Autodesk Fusion 360 part; units mm, degrees
(part 20 of 40)
  line L1487 (51.4118, 42.8386) -> (51.5684, 42.8818) construction
  line L1488 (51.5684, 42.8818) -> (51.7255, 42.9241) construction
  line L1489 (51.7255, 42.9241) -> (51.883, 42.9656) construction
  line L1490 (51.883, 42.9656) -> (52.0409, 43.0063) construction
  line L1491 (52.0409, 43.0063) -> (52.1993, 43.0461) construction
  line L1492 (52.1993, 43.0461) -> (52.3581, 43.085) construction
  line L1493 (52.3581, 43.085) -> (52.5173, 43.1231) construction
  line L1494 (52.5173, 43.1231) -> (52.6769, 43.1604) construction
  line L1495 (52.6769, 43.1604) -> (52.8369, 43.1969) construction
  line L1496 (52.8369, 43.1969) -> (52.9973, 43.2326) construction
  line L1497 (52.9973, 43.2326) -> (53.1581, 43.2674) construction
  line L1498 (53.1581, 43.2674) -> (53.3193, 43.3015) construction
  line L1499 (53.3193, 43.3015) -> (53.4809, 43.3347) construction
  line L1500 (53.4809, 43.3347) -> (53.6428, 43.3672) construction
  line L1501 (53.6428, 43.3672) -> (53.8051, 43.3988) construction
  line L1502 (53.8051, 43.3988) -> (53.9677, 43.4297) construction
  line L1503 (53.9677, 43.4297) -> (54.1307, 43.4597) construction
  line L1504 (54.1307, 43.4597) -> (54.294, 43.489) construction
  line L1505 (54.294, 43.489) -> (54.4577, 43.5175) construction
  line L1506 (54.4577, 43.5175) -> (54.6217, 43.5453) construction
  line L1507 (54.6217, 43.5453) -> (54.7861, 43.5723) construction
  line L1508 (54.7861, 43.5723) -> (54.9508, 43.5984) construction
  line L1509 (54.9508, 43.5984) -> (55.1158, 43.6239) construction
  line L1510 (55.1158, 43.6239) -> (55.2811, 43.6486) construction
  line L1511 (55.2811, 43.6486) -> (55.4467, 43.6725) construction
  line L1512 (55.4467, 43.6725) -> (55.6126, 43.6956) construction
  line L1513 (55.6126, 43.6956) -> (55.7789, 43.718) construction
  line L1514 (55.7789, 43.718) -> (55.9454, 43.7397) construction
  line L1515 (55.9454, 43.7397) -> (56.1122, 43.7606) construction
  line L1516 (56.1122, 43.7606) -> (56.2459, 43.7767) construction
  line L1517 (56.2459, 43.7767) -> (56.3463, 43.7885) construction
  line L1518 (56.3463, 43.7885) -> (56.4133, 43.7962) construction
  line L1519 (56.4133, 43.7962) -> (56.4469, 43.8) construction
  line L1520 (56.0345, -24.1948) -> (56.0628, -24.2071) construction
  line L1521 (56.0628, -24.2071) -> (56.1198, -24.2308) construction
  line L1522 (56.1198, -24.2308) -> (56.2062, -24.264) construction
  line L1523 (56.2062, -24.264) -> (56.3229, -24.3039) construction
  line L1524 (56.3229, -24.3039) -> (56.4711, -24.3478) construction
  line L1525 (56.4711, -24.3478) -> (56.6208, -24.3873) construction
  line L1526 (56.6208, -24.3873) -> (56.7714, -24.4241) construction
  line L1527 (56.7714, -24.4241) -> (56.9226, -24.4595) construction
  line L1528 (56.9226, -24.4595) -> (57.0741, -24.494) construction
  line L1529 (57.0741, -24.494) -> (57.226, -24.5274) construction
  line L1530 (57.226, -24.5274) -> (57.3783, -24.5594) construction
  line L1531 (57.3783, -24.5594) -> (57.5312, -24.5896) construction
  line L1532 (57.5312, -24.5896) -> (57.6848, -24.6176) construction
  line L1533 (57.6848, -24.6176) -> (57.8391, -24.6435) construction
  line L1534 (57.8391, -24.6435) -> (57.994, -24.6674) construction
  line L1535 (57.994, -24.6674) -> (58.1494, -24.6897) construction
  line L1536 (58.1494, -24.6897) -> (58.3052, -24.7105) construction
  line L1537 (58.3052, -24.7105) -> (58.4614, -24.7301) construction
  line L1538 (58.4614, -24.7301) -> (58.6179, -24.7485) construction
  line L1539 (58.6179, -24.7485) -> (58.7747, -24.7658) construction
  line L1540 (58.7747, -24.7658) -> (58.9318, -24.7818) construction
  line L1541 (58.9318, -24.7818) -> (59.0893, -24.7965) construction
  line L1542 (59.0893, -24.7965) -> (59.2471, -24.8098) construction
  line L1543 (59.2471, -24.8098) -> (59.4053, -24.8218) construction
  line L1544 (59.4053, -24.8218) -> (59.5638, -24.8325) construction
  line L1545 (59.5638, -24.8325) -> (59.7226, -24.842) construction
  line L1546 (59.7226, -24.842) -> (59.8817, -24.8504) construction
  line L1547 (59.8817, -24.8504) -> (60.0411, -24.8577) construction
  line L1548 (60.0411, -24.8577) -> (60.2007, -24.8638) construction
  line L1549 (60.2007, -24.8638) -> (60.3605, -24.8689) construction
  line L1550 (60.3605, -24.8689) -> (60.5206, -24.8729) construction
  line L1551 (60.5206, -24.8729) -> (60.6809, -24.8757) construction
  line L1552 (60.6809, -24.8757) -> (60.8415, -24.8776) construction
  line L1553 (60.8415, -24.8776) -> (61.0023, -24.8783) construction
  line L1554 (61.0023, -24.8783) -> (61.1633, -24.878) construction
  line L1555 (61.1633, -24.878) -> (61.3245, -24.8766) construction
  line L1556 (61.3245, -24.8766) -> (61.4859, -24.8742) construction
  line L1557 (61.4859, -24.8742) -> (61.6475, -24.8708) construction
  line L1558 (61.6475, -24.8708) -> (61.8093, -24.8665) construction
  line L1559 (61.8093, -24.8665) -> (61.9712, -24.8611) construction
  line L1560 (61.9712, -24.8611) -> (62.1334, -24.8548) construction
  line L1561 (62.1334, -24.8548) -> (62.2957, -24.8475) construction
  line L1562 (62.2957, -24.8475) -> (62.4581, -24.8392) construction
  line L1563 (62.4581, -24.8392) -> (62.6207, -24.83) construction
  line L1564 (62.6207, -24.83) -> (62.7835, -24.8199) construction
  line L1565 (62.7835, -24.8199) -> (62.9464, -24.8088) construction
  line L1566 (62.9464, -24.8088) -> (63.1095, -24.7967) construction
  line L1567 (63.1095, -24.7967) -> (63.2727, -24.7838) construction
  line L1568 (63.2727, -24.7838) -> (63.436, -24.77) construction
  line L1569 (63.436, -24.77) -> (63.5995, -24.7552) construction
  line L1570 (63.5995, -24.7552) -> (63.7631, -24.7396) construction
  line L1571 (63.7631, -24.7396) -> (63.9268, -24.723) construction
  line L1572 (63.9268, -24.723) -> (64.0906, -24.7056) construction
  line L1573 (64.0906, -24.7056) -> (64.2545, -24.6873) construction
  line L1574 (64.2545, -24.6873) -> (64.4185, -24.6681) construction
  line L1575 (64.4185, -24.6681) -> (64.5826, -24.648) construction
  line L1576 (64.5826, -24.648) -> (64.7468, -24.6271) construction
  line L1577 (64.7468, -24.6271) -> (64.9111, -24.6054) construction
  line L1578 (64.9111, -24.6054) -> (65.0755, -24.5828) construction
  line L1579 (65.0755, -24.5828) -> (65.24, -24.5593) construction
  line L1580 (65.24, -24.5593) -> (65.4046, -24.535) construction
  line L1581 (65.4046, -24.535) -> (65.5692, -24.5098) construction
  line L1582 (65.5692, -24.5098) -> (65.734, -24.4839) construction
  line L1583 (65.734, -24.4839) -> (65.8987, -24.4571) construction
  line L1584 (65.8987, -24.4571) -> (66.0636, -24.4294) construction
  line L1585 (66.0636, -24.4294) -> (66.2285, -24.401) construction
  line L1586 (66.2285, -24.401) -> (66.3935, -24.3718) construction
  line L1587 (66.3935, -24.3718) -> (66.5585, -24.3417) construction
  line L1588 (66.5585, -24.3417) -> (66.7236, -24.3108) construction
  line L1589 (66.7236, -24.3108) -> (66.8887, -24.2792) construction
  line L1590 (66.8887, -24.2792) -> (67.0208, -24.2532) construction
  line L1591 (67.0208, -24.2532) -> (67.1199, -24.2334) construction
  line L1592 (67.1199, -24.2334) -> (67.186, -24.22) construction
  line L1593 (67.186, -24.22) -> (67.2191, -24.2132) construction
  line L1594 (52.5103, -31.1115) -> (52.5368, -31.1272) construction
  line L1595 (52.5368, -31.1272) -> (52.5895, -31.1594) construction
  line L1596 (52.5895, -31.1594) -> (52.6672, -31.2097) construction
  line L1597 (52.6672, -31.2097) -> (52.7681, -31.2807) construction
  line L1598 (52.7681, -31.2807) -> (52.8906, -31.3748) construction
  line L1599 (52.8906, -31.3748) -> (53.0106, -31.4727) construction
  line L1600 (53.0106, -31.4727) -> (53.1289, -31.5729) construction
  line L1601 (53.1289, -31.5729) -> (53.2464, -31.6744) construction
  line L1602 (53.2464, -31.6744) -> (53.3634, -31.7767) construction
  line L1603 (53.3634, -31.7767) -> (53.4797, -31.88) construction
  line L1604 (53.4797, -31.88) -> (53.5951, -31.9844) construction
  line L1605 (53.5951, -31.9844) -> (53.7094, -32.0903) construction
  line L1606 (53.7094, -32.0903) -> (53.8224, -32.1981) construction
  line L1607 (53.8224, -32.1981) -> (53.934, -32.3077) construction
  line L1608 (53.934, -32.3077) -> (54.0444, -32.419) construction
  line L1609 (54.0444, -32.419) -> (54.1537, -32.5316) construction
  line L1610 (54.1537, -32.5316) -> (54.2622, -32.6455) construction
  line L1611 (54.2622, -32.6455) -> (54.3698, -32.7603) construction
  line L1612 (54.3698, -32.7603) -> (54.4767, -32.876) construction
  line L1613 (54.4767, -32.876) -> (54.5828, -32.9927) construction
  line L1614 (54.5828, -32.9927) -> (54.6881, -33.1105) construction
  line L1615 (54.6881, -33.1105) -> (54.7926, -33.2292) construction
  line L1616 (54.7926, -33.2292) -> (54.8961, -33.3491) construction
  line L1617 (54.8961, -33.3491) -> (54.9988, -33.47) construction
  line L1618 (54.9988, -33.47) -> (55.1007, -33.5919) construction
  line L1619 (55.1007, -33.5919) -> (55.2017, -33.7148) construction
  line L1620 (55.2017, -33.7148) -> (55.302, -33.8386) construction
  line L1621 (55.302, -33.8386) -> (55.4015, -33.9633) construction
  line L1622 (55.4015, -33.9633) -> (55.5003, -34.0888) construction
  line L1623 (55.5003, -34.0888) -> (55.5984, -34.2151) construction
  line L1624 (55.5984, -34.2151) -> (55.6957, -34.3423) construction
  line L1625 (55.6957, -34.3423) -> (55.7923, -34.4703) construction
  line L1626 (55.7923, -34.4703) -> (55.8881, -34.5991) construction
  line L1627 (55.8881, -34.5991) -> (55.9832, -34.7288) construction
  line L1628 (55.9832, -34.7288) -> (56.0776, -34.8592) construction
  line L1629 (56.0776, -34.8592) -> (56.1712, -34.9905) construction
  line L1630 (56.1712, -34.9905) -> (56.2642, -35.1224) construction
  line L1631 (56.2642, -35.1224) -> (56.3564, -35.2552) construction
  line L1632 (56.3564, -35.2552) -> (56.448, -35.3886) construction
  line L1633 (56.448, -35.3886) -> (56.5388, -35.5228) construction
  line L1634 (56.5388, -35.5228) -> (56.629, -35.6577) construction
  line L1635 (56.629, -35.6577) -> (56.7185, -35.7933) construction
  line L1636 (56.7185, -35.7933) -> (56.8073, -35.9295) construction
  line L1637 (56.8073, -35.9295) -> (56.8955, -36.0665) construction
  line L1638 (56.8955, -36.0665) -> (56.9829, -36.2042) construction
  line L1639 (56.9829, -36.2042) -> (57.0697, -36.3425) construction
  line L1640 (57.0697, -36.3425) -> (57.1558, -36.4815) construction
  line L1641 (57.1558, -36.4815) -> (57.2413, -36.6211) construction
  line L1642 (57.2413, -36.6211) -> (57.3261, -36.7614) construction
  line L1643 (57.3261, -36.7614) -> (57.4102, -36.9023) construction
  line L1644 (57.4102, -36.9023) -> (57.4937, -37.0438) construction
  line L1645 (57.4937, -37.0438) -> (57.5765, -37.186) construction
  line L1646 (57.5765, -37.186) -> (57.6587, -37.3288) construction
  line L1647 (57.6587, -37.3288) -> (57.7403, -37.4721) construction
  line L1648 (57.7403, -37.4721) -> (57.8212, -37.6161) construction
  line L1649 (57.8212, -37.6161) -> (57.9014, -37.7607) construction
  line L1650 (57.9014, -37.7607) -> (57.981, -37.9058) construction
  line L1651 (57.981, -37.9058) -> (58.06, -38.0515) construction
  line L1652 (58.06, -38.0515) -> (58.1383, -38.1978) construction
  line L1653 (58.1383, -38.1978) -> (58.216, -38.3447) construction
  line L1654 (58.216, -38.3447) -> (58.2931, -38.4921) construction
  line L1655 (58.2931, -38.4921) -> (58.3695, -38.6401) construction
  line L1656 (58.3695, -38.6401) -> (58.4453, -38.7886) construction
  line L1657 (58.4453, -38.7886) -> (58.5205, -38.9377) construction
  line L1658 (58.5205, -38.9377) -> (58.595, -39.0873) construction
  line L1659 (58.595, -39.0873) -> (58.669, -39.2374) construction
  line L1660 (58.669, -39.2374) -> (58.7423, -39.3881) construction
  line L1661 (58.7423, -39.3881) -> (58.8149, -39.5393) construction
  line L1662 (58.8149, -39.5393) -> (58.887, -39.6909) construction
  line L1663 (58.887, -39.6909) -> (58.9584, -39.8431) construction
  line L1664 (58.9584, -39.8431) -> (59.0151, -39.9653) construction
  line L1665 (59.0151, -39.9653) -> (59.0573, -40.0572) construction
  line L1666 (59.0573, -40.0572) -> (59.0853, -40.1185) construction
  line L1667 (59.0853, -40.1185) -> (59.0993, -40.1492) construction
  line L1668 (-13.3622, -59.5542) -> (-13.369, -59.5843) construction
  line L1669 (-13.369, -59.5843) -> (-13.3833, -59.6444) construction
  line L1670 (-13.3833, -59.6444) -> (-13.4071, -59.7338) construction
  line L1671 (-13.4071, -59.7338) -> (-13.4435, -59.8517) construction
  line L1672 (-13.4435, -59.8517) -> (-13.4951, -59.9973) construction
  line L1673 (-13.4951, -59.9973) -> (-13.5511, -60.1416) construction
  line L1674 (-13.5511, -60.1416) -> (-13.6099, -60.2852) construction
  line L1675 (-13.6099, -60.2852) -> (-13.6701, -60.4283) construction
  line L1676 (-13.6701, -60.4283) -> (-13.7313, -60.5711) construction
  line L1677 (-13.7313, -60.5711) -> (-13.7935, -60.7136) construction
  line L1678 (-13.7935, -60.7136) -> (-13.8571, -60.8557) construction
  line L1679 (-13.8571, -60.8557) -> (-13.9226, -60.9971) construction
  line L1680 (-13.9226, -60.9971) -> (-13.9902, -61.1379) construction
  line L1681 (-13.9902, -61.1379) -> (-14.06, -61.2779) construction
  line L1682 (-14.06, -61.2779) -> (-14.1316, -61.4173) construction
  line L1683 (-14.1316, -61.4173) -> (-14.205, -61.5561) construction
  line L1684 (-14.205, -61.5561) -> (-14.2797, -61.6944) construction
  line L1685 (-14.2797, -61.6944) -> (-14.3557, -61.8322) construction
  line L1686 (-14.3557, -61.8322) -> (-14.4327, -61.9697) construction
  line L1687 (-14.4327, -61.9697) -> (-14.5109, -62.1067) construction
  line L1688 (-14.5109, -62.1067) -> (-14.5904, -62.2432) construction
  line L1689 (-14.5904, -62.2432) -> (-14.6711, -62.3792) construction
  line L1690 (-14.6711, -62.3792) -> (-14.753, -62.5148) construction
  line L1691 (-14.753, -62.5148) -> (-14.8363, -62.6498) construction
  line L1692 (-14.8363, -62.6498) -> (-14.9208, -62.7843) construction
  line L1693 (-14.9208, -62.7843) -> (-15.0064, -62.9184) construction
  line L1694 (-15.0064, -62.9184) -> (-15.0932, -63.052) construction
  line L1695 (-15.0932, -63.052) -> (-15.181, -63.1852) construction
  line L1696 (-15.181, -63.1852) -> (-15.2698, -63.318) construction
  line L1697 (-15.2698, -63.318) -> (-15.3597, -63.4503) construction
  line L1698 (-15.3597, -63.4503) -> (-15.4506, -63.5821) construction
  line L1699 (-15.4506, -63.5821) -> (-15.5425, -63.7135) construction
  line L1700 (-15.5425, -63.7135) -> (-15.6354, -63.8445) construction
  line L1701 (-15.6354, -63.8445) -> (-15.7293, -63.975) construction
  line L1702 (-15.7293, -63.975) -> (-15.8242, -64.105) construction
  line L1703 (-15.8242, -64.105) -> (-15.92, -64.2346) construction
  line L1704 (-15.92, -64.2346) -> (-16.0168, -64.3638) construction
  line L1705 (-16.0168, -64.3638) -> (-16.1146, -64.4926) construction
  line L1706 (-16.1146, -64.4926) -> (-16.2132, -64.6209) construction
  line L1707 (-16.2132, -64.6209) -> (-16.3127, -64.7488) construction
  line L1708 (-16.3127, -64.7488) -> (-16.4131, -64.8762) construction
  line L1709 (-16.4131, -64.8762) -> (-16.5144, -65.0032) construction
  line L1710 (-16.5144, -65.0032) -> (-16.6166, -65.1298) construction
  line L1711 (-16.6166, -65.1298) -> (-16.7196, -65.256) construction
  line L1712 (-16.7196, -65.256) -> (-16.8235, -65.3817) construction
  line L1713 (-16.8235, -65.3817) -> (-16.9283, -65.507) construction
  line L1714 (-16.9283, -65.507) -> (-17.0338, -65.6318) construction
  line L1715 (-17.0338, -65.6318) -> (-17.1402, -65.7562) construction
  line L1716 (-17.1402, -65.7562) -> (-17.2474, -65.8802) construction
  line L1717 (-17.2474, -65.8802) -> (-17.3555, -66.0038) construction
  line L1718 (-17.3555, -66.0038) -> (-17.4643, -66.1269) construction
  line L1719 (-17.4643, -66.1269) -> (-17.5739, -66.2497) construction
  line L1720 (-17.5739, -66.2497) -> (-17.6842, -66.3719) construction
  line L1721 (-17.6842, -66.3719) -> (-17.7954, -66.4938) construction
  line L1722 (-17.7954, -66.4938) -> (-17.9073, -66.6152) construction
  line L1723 (-17.9073, -66.6152) -> (-18.02, -66.7362) construction
  line L1724 (-18.02, -66.7362) -> (-18.1335, -66.8568) construction
  line L1725 (-18.1335, -66.8568) -> (-18.2477, -66.9769) construction
  line L1726 (-18.2477, -66.9769) -> (-18.3626, -67.0966) construction
  line L1727 (-18.3626, -67.0966) -> (-18.4782, -67.2159) construction
  line L1728 (-18.4782, -67.2159) -> (-18.5946, -67.3347) construction
  line L1729 (-18.5946, -67.3347) -> (-18.7118, -67.4531) construction
  line L1730 (-18.7118, -67.4531) -> (-18.8296, -67.5711) construction
  line L1731 (-18.8296, -67.5711) -> (-18.9481, -67.6887) construction
  line L1732 (-18.9481, -67.6887) -> (-19.0674, -67.8058) construction
  line L1733 (-19.0674, -67.8058) -> (-19.1873, -67.9225) construction
  line L1734 (-19.1873, -67.9225) -> (-19.3079, -68.0388) construction
  line L1735 (-19.3079, -68.0388) -> (-19.4293, -68.1546) construction
  line L1736 (-19.4293, -68.1546) -> (-19.5512, -68.27) construction
  line L1737 (-19.5512, -68.27) -> (-19.6739, -68.385) construction
  line L1738 (-19.6739, -68.385) -> (-19.7726, -68.4767) construction
  line L1739 (-19.7726, -68.4767) -> (-19.8469, -68.5452) construction
  line L1740 (-19.8469, -68.5452) -> (-19.8966, -68.5908) construction
  line L1741 (-19.8966, -68.5908) -> (-19.9215, -68.6136) construction
  line L1742 (-45.8153, 40.3263) -> (-45.8385, 40.3467) construction
  line L1743 (-45.8385, 40.3467) -> (-45.8854, 40.3868) construction
  line L1744 (-45.8854, 40.3868) -> (-45.9573, 40.4451) construction
  line L1745 (-45.9573, 40.4451) -> (-46.056, 40.5192) construction
  line L1746 (-46.056, 40.5192) -> (-46.1833, 40.6066) construction
  line L1747 (-46.1833, 40.6066) -> (-46.3135, 40.6904) construction
  line L1748 (-46.3135, 40.6904) -> (-46.4454, 40.772) construction
  line L1749 (-46.4454, 40.772) -> (-46.5782, 40.8524) construction
  line L1750 (-46.5782, 40.8524) -> (-46.7117, 40.932) construction
  line L1751 (-46.7117, 40.932) -> (-46.8458, 41.0107) construction
  line L1752 (-46.8458, 41.0107) -> (-46.9807, 41.0883) construction
  line L1753 (-46.9807, 41.0883) -> (-47.1168, 41.1642) construction
  line L1754 (-47.1168, 41.1642) -> (-47.2543, 41.2383) construction
  line L1755 (-47.2543, 41.2383) -> (-47.393, 41.3106) construction
  line L1756 (-47.393, 41.3106) -> (-47.5329, 41.3813) construction
  line L1757 (-47.5329, 41.3813) -> (-47.6738, 41.4504) construction
  line L1758 (-47.6738, 41.4504) -> (-47.8156, 41.5184) construction
  line L1759 (-47.8156, 41.5184) -> (-47.9581, 41.5853) construction
  line L1760 (-47.9581, 41.5853) -> (-48.1012, 41.6512) construction
  line L1761 (-48.1012, 41.6512) -> (-48.245, 41.716) construction
  line L1762 (-48.245, 41.716) -> (-48.3895, 41.7798) construction
  line L1763 (-48.3895, 41.7798) -> (-48.5347, 41.8424) construction
  line L1764 (-48.5347, 41.8424) -> (-48.6807, 41.9039) construction
  line L1765 (-48.6807, 41.9039) -> (-48.8274, 41.9642) construction
  line L1766 (-48.8274, 41.9642) -> (-48.9749, 42.0234) construction
  line L1767 (-48.9749, 42.0234) -> (-49.123, 42.0815) construction
  line L1768 (-49.123, 42.0815) -> (-49.2717, 42.1386) construction
  line L1769 (-49.2717, 42.1386) -> (-49.421, 42.1947) construction
  line L1770 (-49.421, 42.1947) -> (-49.5709, 42.2499) construction
  line L1771 (-49.5709, 42.2499) -> (-49.7214, 42.3041) construction
  line L1772 (-49.7214, 42.3041) -> (-49.8724, 42.3574) construction
  line L1773 (-49.8724, 42.3574) -> (-50.024, 42.4097) construction
  line L1774 (-50.024, 42.4097) -> (-50.1761, 42.461) construction
  line L1775 (-50.1761, 42.461) -> (-50.3288, 42.5114) construction
  line L1776 (-50.3288, 42.5114) -> (-50.482, 42.5608) construction
  line L1777 (-50.482, 42.5608) -> (-50.6358, 42.6094) construction
  line L1778 (-50.6358, 42.6094) -> (-50.79, 42.657) construction
  line L1779 (-50.79, 42.657) -> (-50.9447, 42.7037) construction
  line L1780 (-50.9447, 42.7037) -> (-51.0999, 42.7495) construction
  line L1781 (-51.0999, 42.7495) -> (-51.2556, 42.7945) construction
  line L1782 (-51.2556, 42.7945) -> (-51.4118, 42.8386) construction
  line L1783 (-51.4118, 42.8386) -> (-51.5684, 42.8818) construction
  line L1784 (-51.5684, 42.8818) -> (-51.7255, 42.9241) construction
  line L1785 (-51.7255, 42.9241) -> (-51.883, 42.9656) construction
  line L1786 (-51.883, 42.9656) -> (-52.0409, 43.0063) construction
  line L1787 (-52.0409, 43.0063) -> (-52.1993, 43.0461) construction
  line L1788 (-52.1993, 43.0461) -> (-52.3581, 43.085) construction
  line L1789 (-52.3581, 43.085) -> (-52.5173, 43.1231) construction
  line L1790 (-52.5173, 43.1231) -> (-52.6769, 43.1604) construction
  line L1791 (-52.6769, 43.1604) -> (-52.8369, 43.1969) construction
  line L1792 (-52.8369, 43.1969) -> (-52.9973, 43.2326) construction
  line L1793 (-52.9973, 43.2326) -> (-53.1581, 43.2674) construction
  line L1794 (-53.1581, 43.2674) -> (-53.3193, 43.3015) construction
  line L1795 (-53.3193, 43.3015) -> (-53.4809, 43.3347) construction
  line L1796 (-53.4809, 43.3347) -> (-53.6428, 43.3672) construction
  line L1797 (-53.6428, 43.3672) -> (-53.8051, 43.3988) construction
  line L1798 (-53.8051, 43.3988) -> (-53.9677, 43.4297) construction
  line L1799 (-53.9677, 43.4297) -> (-54.1307, 43.4597) construction
  line L1800 (-54.1307, 43.4597) -> (-54.294, 43.489) construction
  line L1801 (-54.294, 43.489) -> (-54.4577, 43.5175) construction
  line L1802 (-54.4577, 43.5175) -> (-54.6217, 43.5453) construction
  line L1803 (-54.6217, 43.5453) -> (-54.7861, 43.5723) construction
  line L1804 (-54.7861, 43.5723) -> (-54.9508, 43.5984) construction
  line L1805 (-54.9508, 43.5984) -> (-55.1158, 43.6239) construction
  line L1806 (-55.1158, 43.6239) -> (-55.2811, 43.6486) construction
  line L1807 (-55.2811, 43.6486) -> (-55.4467, 43.6725) construction
  line L1808 (-55.4467, 43.6725) -> (-55.6126, 43.6956) construction
  line L1809 (-55.6126, 43.6956) -> (-55.7789, 43.718) construction
  line L1810 (-55.7789, 43.718) -> (-55.9454, 43.7397) construction
  line L1811 (-55.9454, 43.7397) -> (-56.1122, 43.7606) construction
  line L1812 (-56.1122, 43.7606) -> (-56.2459, 43.7767) construction
  line L1813 (-56.2459, 43.7767) -> (-56.3463, 43.7885) construction
  line L1814 (-56.3463, 43.7885) -> (-56.4133, 43.7962) construction
  line L1815 (-56.4133, 43.7962) -> (-56.4469, 43.8) construction
  line L1816 (59.5542, 13.3622) -> (59.5843, 13.369) construction
  line L1817 (59.5843, 13.369) -> (59.6444, 13.3833) construction
  line L1818 (59.6444, 13.3833) -> (59.7338, 13.4071) construction
  line L1819 (59.7338, 13.4071) -> (59.8517, 13.4435) construction
  line L1820 (59.8517, 13.4435) -> (59.9973, 13.4951) construction
  line L1821 (59.9973, 13.4951) -> (60.1416, 13.5511) construction
  line L1822 (60.1416, 13.5511) -> (60.2852, 13.6099) construction
  line L1823 (60.2852, 13.6099) -> (60.4283, 13.6701) construction
  line L1824 (60.4283, 13.6701) -> (60.5711, 13.7313) construction
  line L1825 (60.5711, 13.7313) -> (60.7136, 13.7935) construction
  line L1826 (60.7136, 13.7935) -> (60.8557, 13.8571) construction
  line L1827 (60.8557, 13.8571) -> (60.9971, 13.9226) construction
  line L1828 (60.9971, 13.9226) -> (61.1379, 13.9902) construction
  line L1829 (61.1379, 13.9902) -> (61.2779, 14.06) construction
  line L1830 (61.2779, 14.06) -> (61.4173, 14.1316) construction
  line L1831 (61.4173, 14.1316) -> (61.5561, 14.205) construction
  line L1832 (61.5561, 14.205) -> (61.6944, 14.2797) construction
  line L1833 (61.6944, 14.2797) -> (61.8322, 14.3557) construction
  line L1834 (61.8322, 14.3557) -> (61.9697, 14.4327) construction
  line L1835 (61.9697, 14.4327) -> (62.1067, 14.5109) construction
  line L1836 (62.1067, 14.5109) -> (62.2432, 14.5904) construction
  line L1837 (62.2432, 14.5904) -> (62.3792, 14.6711) construction
  line L1838 (62.3792, 14.6711) -> (62.5148, 14.753) construction
  line L1839 (62.5148, 14.753) -> (62.6498, 14.8363) construction
  line L1840 (62.6498, 14.8363) -> (62.7843, 14.9208) construction
  line L1841 (62.7843, 14.9208) -> (62.9184, 15.0064) construction
  line L1842 (62.9184, 15.0064) -> (63.052, 15.0932) construction
  line L1843 (63.052, 15.0932) -> (63.1852, 15.181) construction
  line L1844 (63.1852, 15.181) -> (63.318, 15.2698) construction
  line L1845 (63.318, 15.2698) -> (63.4503, 15.3597) construction
  line L1846 (63.4503, 15.3597) -> (63.5821, 15.4506) construction
  line L1847 (63.5821, 15.4506) -> (63.7135, 15.5425) construction
  line L1848 (63.7135, 15.5425) -> (63.8445, 15.6354) construction
  line L1849 (63.8445, 15.6354) -> (63.975, 15.7293) construction
  line L1850 (63.975, 15.7293) -> (64.105, 15.8242) construction
  line L1851 (64.105, 15.8242) -> (64.2346, 15.92) construction
  line L1852 (64.2346, 15.92) -> (64.3638, 16.0168) construction
  line L1853 (64.3638, 16.0168) -> (64.4926, 16.1146) construction
  line L1854 (64.4926, 16.1146) -> (64.6209, 16.2132) construction
  line L1855 (64.6209, 16.2132) -> (64.7488, 16.3127) construction
  line L1856 (64.7488, 16.3127) -> (64.8762, 16.4131) construction
  line L1857 (64.8762, 16.4131) -> (65.0032, 16.5144) construction
  line L1858 (65.0032, 16.5144) -> (65.1298, 16.6166) construction
  line L1859 (65.1298, 16.6166) -> (65.256, 16.7196) construction
  line L1860 (65.256, 16.7196) -> (65.3817, 16.8235) construction
  line L1861 (65.3817, 16.8235) -> (65.507, 16.9283) construction
  line L1862 (65.507, 16.9283) -> (65.6318, 17.0338) construction
  line L1863 (65.6318, 17.0338) -> (65.7562, 17.1402) construction
  line L1864 (65.7562, 17.1402) -> (65.8802, 17.2474) construction
  line L1865 (65.8802, 17.2474) -> (66.0038, 17.3555) construction
  line L1866 (66.0038, 17.3555) -> (66.1269, 17.4643) construction
  line L1867 (66.1269, 17.4643) -> (66.2497, 17.5739) construction
  line L1868 (66.2497, 17.5739) -> (66.3719, 17.6842) construction
  line L1869 (66.3719, 17.6842) -> (66.4938, 17.7954) construction
  line L1870 (66.4938, 17.7954) -> (66.6152, 17.9073) construction
  line L1871 (66.6152, 17.9073) -> (66.7362, 18.02) construction
  line L1872 (66.7362, 18.02) -> (66.8568, 18.1335) construction
  line L1873 (66.8568, 18.1335) -> (66.9769, 18.2477) construction
  line L1874 (66.9769, 18.2477) -> (67.0966, 18.3626) construction
  line L1875 (67.0966, 18.3626) -> (67.2159, 18.4782) construction
  line L1876 (67.2159, 18.4782) -> (67.3347, 18.5946) construction
  line L1877 (67.3347, 18.5946) -> (67.4531, 18.7118) construction
  line L1878 (67.4531, 18.7118) -> (67.5711, 18.8296) construction
  line L1879 (67.5711, 18.8296) -> (67.6887, 18.9481) construction
  line L1880 (67.6887, 18.9481) -> (67.8058, 19.0674) construction
  line L1881 (67.8058, 19.0674) -> (67.9225, 19.1873) construction
  line L1882 (67.9225, 19.1873) -> (68.0388, 19.3079) construction
  line L1883 (68.0388, 19.3079) -> (68.1546, 19.4293) construction
  line L1884 (68.1546, 19.4293) -> (68.27, 19.5512) construction
  line L1885 (68.27, 19.5512) -> (68.385, 19.6739) construction
  line L1886 (68.385, 19.6739) -> (68.4767, 19.7726) construction
  line L1887 (68.4767, 19.7726) -> (68.5452, 19.8469) construction
  line L1888 (68.5452, 19.8469) -> (68.5908, 19.8966) construction
  line L1889 (68.5908, 19.8966) -> (68.6136, 19.9215) construction
  line L1890 (-60.7685, -5.6951) -> (-60.7993, -5.6979) construction
  line L1891 (-60.7993, -5.6979) -> (-60.8609, -5.7029) construction
  line L1892 (-60.8609, -5.7029) -> (-60.9533, -5.7078) construction
  line L1893 (-60.9533, -5.7078) -> (-61.0766, -5.7097) construction
  line L1894 (-61.0766, -5.7097) -> (-61.231, -5.7056) construction
  line L1895 (-61.231, -5.7056) -> (-61.3856, -5.6969) construction
  line L1896 (-61.3856, -5.6969) -> (-61.5403, -5.6854) construction
  line L1897 (-61.5403, -5.6854) -> (-61.695, -5.6723) construction
  line L1898 (-61.695, -5.6723) -> (-61.8498, -5.6583) construction
  line L1899 (-61.8498, -5.6583) -> (-62.0045, -5.6431) construction
  line L1900 (-62.0045, -5.6431) -> (-62.1593, -5.6265) construction
  line L1901 (-62.1593, -5.6265) -> (-62.314, -5.608) construction
  line L1902 (-62.314, -5.608) -> (-62.4688, -5.5871) construction
  line L1903 (-62.4688, -5.5871) -> (-62.6235, -5.5641) construction
  line L1904 (-62.6235, -5.5641) -> (-62.7782, -5.539) construction
  line L1905 (-62.7782, -5.539) -> (-62.9329, -5.5121) construction
  line L1906 (-62.9329, -5.5121) -> (-63.0875, -5.4838) construction
  line L1907 (-63.0875, -5.4838) -> (-63.2421, -5.4542) construction
  line L1908 (-63.2421, -5.4542) -> (-63.3966, -5.4233) construction
  line L1909 (-63.3966, -5.4233) -> (-63.5511, -5.3913) construction
  line L1910 (-63.5511, -5.3913) -> (-63.7055, -5.3579) construction
  line L1911 (-63.7055, -5.3579) -> (-63.8598, -5.3232) construction
  line L1912 (-63.8598, -5.3232) -> (-64.014, -5.2871) construction
  line L1913 (-64.014, -5.2871) -> (-64.1682, -5.2497) construction
  line L1914 (-64.1682, -5.2497) -> (-64.3222, -5.2109) construction
  line L1915 (-64.3222, -5.2109) -> (-64.4762, -5.1709) construction
  line L1916 (-64.4762, -5.1709) -> (-64.6301, -5.1297) construction
  line L1917 (-64.6301, -5.1297) -> (-64.7839, -5.0873) construction
  line L1918 (-64.7839, -5.0873) -> (-64.9376, -5.0439) construction
  line L1919 (-64.9376, -5.0439) -> (-65.0912, -4.9993) construction
  line L1920 (-65.0912, -4.9993) -> (-65.2447, -4.9536) construction
  line L1921 (-65.2447, -4.9536) -> (-65.398, -4.9068) construction
  line L1922 (-65.398, -4.9068) -> (-65.5513, -4.8589) construction
  line L1923 (-65.5513, -4.8589) -> (-65.7044, -4.8099) construction
  line L1924 (-65.7044, -4.8099) -> (-65.8574, -4.7599) construction
  line L1925 (-65.8574, -4.7599) -> (-66.0103, -4.7087) construction
  line L1926 (-66.0103, -4.7087) -> (-66.1631, -4.6566) construction
  line L1927 (-66.1631, -4.6566) -> (-66.3158, -4.6035) construction
  line L1928 (-66.3158, -4.6035) -> (-66.4683, -4.5493) construction
  line L1929 (-66.4683, -4.5493) -> (-66.6206, -4.4942) construction
  line L1930 (-66.6206, -4.4942) -> (-66.7729, -4.438) construction
  line L1931 (-66.7729, -4.438) -> (-66.925, -4.381) construction
  line L1932 (-66.925, -4.381) -> (-67.077, -4.3229) construction
  line L1933 (-67.077, -4.3229) -> (-67.2288, -4.2639) construction
  line L1934 (-67.2288, -4.2639) -> (-67.3804, -4.2039) construction
  line L1935 (-67.3804, -4.2039) -> (-67.532, -4.143) construction
  line L1936 (-67.532, -4.143) -> (-67.6833, -4.0812) construction
  line L1937 (-67.6833, -4.0812) -> (-67.8345, -4.0185) construction
  line L1938 (-67.8345, -4.0185) -> (-67.9856, -3.9548) construction
  line L1939 (-67.9856, -3.9548) -> (-68.1365, -3.8903) construction
  line L1940 (-68.1365, -3.8903) -> (-68.2872, -3.8249) construction
  line L1941 (-68.2872, -3.8249) -> (-68.4378, -3.7585) construction
  line L1942 (-68.4378, -3.7585) -> (-68.5882, -3.6913) construction
  line L1943 (-68.5882, -3.6913) -> (-68.7384, -3.6233) construction
  line L1944 (-68.7384, -3.6233) -> (-68.8885, -3.5543) construction
  line L1945 (-68.8885, -3.5543) -> (-69.0384, -3.4846) construction
  line L1946 (-69.0384, -3.4846) -> (-69.1881, -3.4139) construction
  line L1947 (-69.1881, -3.4139) -> (-69.3376, -3.3425) construction
  line L1948 (-69.3376, -3.3425) -> (-69.487, -3.2701) construction
  line L1949 (-69.487, -3.2701) -> (-69.6362, -3.197) construction
  line L1950 (-69.6362, -3.197) -> (-69.7852, -3.123) construction
  line L1951 (-69.7852, -3.123) -> (-69.934, -3.0482) construction
  line L1952 (-69.934, -3.0482) -> (-70.0826, -2.9726) construction
  line L1953 (-70.0826, -2.9726) -> (-70.2311, -2.8962) construction
  line L1954 (-70.2311, -2.8962) -> (-70.3793, -2.819) construction
  line L1955 (-70.3793, -2.819) -> (-70.5274, -2.741) construction
  line L1956 (-70.5274, -2.741) -> (-70.6752, -2.6622) construction
  line L1957 (-70.6752, -2.6622) -> (-70.8229, -2.5826) construction
  line L1958 (-70.8229, -2.5826) -> (-70.9703, -2.5023) construction
  line L1959 (-70.9703, -2.5023) -> (-71.1176, -2.4211) construction
  line L1960 (-71.1176, -2.4211) -> (-71.2352, -2.3556) construction
  line L1961 (-71.2352, -2.3556) -> (-71.3234, -2.3061) construction
  line L1962 (-71.3234, -2.3061) -> (-71.3821, -2.2729) construction
  line L1963 (-71.3821, -2.2729) -> (-71.4115, -2.2563) construction
  line L1964 (56.0345, 24.1948) -> (56.0628, 24.2071) construction
  line L1965 (56.0628, 24.2071) -> (56.1198, 24.2308) construction
  line L1966 (56.1198, 24.2308) -> (56.2062, 24.264) construction
  line L1967 (56.2062, 24.264) -> (56.3229, 24.3039) construction
  line L1968 (56.3229, 24.3039) -> (56.4711, 24.3478) construction
  line L1969 (56.4711, 24.3478) -> (56.6208, 24.3873) construction
  line L1970 (56.6208, 24.3873) -> (56.7714, 24.4241) construction
  line L1971 (56.7714, 24.4241) -> (56.9226, 24.4595) construction
  line L1972 (56.9226, 24.4595) -> (57.0741, 24.494) construction
  line L1973 (57.0741, 24.494) -> (57.226, 24.5274) construction
  line L1974 (57.226, 24.5274) -> (57.3783, 24.5594) construction
  line L1975 (57.3783, 24.5594) -> (57.5312, 24.5896) construction
  line L1976 (57.5312, 24.5896) -> (57.6848, 24.6176) construction
  line L1977 (57.6848, 24.6176) -> (57.8391, 24.6435) construction
  line L1978 (57.8391, 24.6435) -> (57.994, 24.6674) construction
  line L1979 (57.994, 24.6674) -> (58.1494, 24.6897) construction
  line L1980 (58.1494, 24.6897) -> (58.3052, 24.7105) construction
  line L1981 (58.3052, 24.7105) -> (58.4614, 24.7301) construction
  line L1982 (58.4614, 24.7301) -> (58.6179, 24.7485) construction
  line L1983 (58.6179, 24.7485) -> (58.7747, 24.7658) construction
  line L1984 (58.7747, 24.7658) -> (58.9318, 24.7818) construction
  line L1985 (58.9318, 24.7818) -> (59.0893, 24.7965) construction
  line L1986 (59.0893, 24.7965) -> (59.2471, 24.8098) construction
  line L1987 (59.2471, 24.8098) -> (59.4053, 24.8218) construction
  line L1988 (59.4053, 24.8218) -> (59.5638, 24.8325) construction
  line L1989 (59.5638, 24.8325) -> (59.7226, 24.842) construction
  line L1990 (59.7226, 24.842) -> (59.8817, 24.8504) construction
  line L1991 (59.8817, 24.8504) -> (60.0411, 24.8577) construction
  line L1992 (60.0411, 24.8577) -> (60.2007, 24.8638) construction
  line L1993 (60.2007, 24.8638) -> (60.3605, 24.8689) construction
  line L1994 (60.3605, 24.8689) -> (60.5206, 24.8729) construction
  line L1995 (60.5206, 24.8729) -> (60.6809, 24.8757) construction
  line L1996 (60.6809, 24.8757) -> (60.8415, 24.8776) construction
  line L1997 (60.8415, 24.8776) -> (61.0023, 24.8783) construction
  line L1998 (61.0023, 24.8783) -> (61.1633, 24.878) construction
  line L1999 (61.1633, 24.878) -> (61.3245, 24.8766) construction
  line L2000 (61.3245, 24.8766) -> (61.4859, 24.8742) construction
  line L2001 (61.4859, 24.8742) -> (61.6475, 24.8708) construction
  line L2002 (61.6475, 24.8708) -> (61.8093, 24.8665) construction
  line L2003 (61.8093, 24.8665) -> (61.9712, 24.8611) construction
  line L2004 (61.9712, 24.8611) -> (62.1334, 24.8548) construction
  line L2005 (62.1334, 24.8548) -> (62.2957, 24.8475) construction
  line L2006 (62.2957, 24.8475) -> (62.4581, 24.8392) construction
  line L2007 (62.4581, 24.8392) -> (62.6207, 24.83) construction
  line L2008 (62.6207, 24.83) -> (62.7835, 24.8199) construction
  line L2009 (62.7835, 24.8199) -> (62.9464, 24.8088) construction
  line L2010 (62.9464, 24.8088) -> (63.1095, 24.7967) construction
  line L2011 (63.1095, 24.7967) -> (63.2727, 24.7838) construction
  line L2012 (63.2727, 24.7838) -> (63.436, 24.77) construction
  line L2013 (63.436, 24.77) -> (63.5995, 24.7552) construction
  line L2014 (63.5995, 24.7552) -> (63.7631, 24.7396) construction
  line L2015 (63.7631, 24.7396) -> (63.9268, 24.723) construction
  line L2016 (63.9268, 24.723) -> (64.0906, 24.7056) construction
  line L2017 (64.0906, 24.7056) -> (64.2545, 24.6873) construction
  line L2018 (64.2545, 24.6873) -> (64.4185, 24.6681) construction
  line L2019 (64.4185, 24.6681) -> (64.5826, 24.648) construction
  line L2020 (64.5826, 24.648) -> (64.7468, 24.6271) construction
  line L2021 (64.7468, 24.6271) -> (64.9111, 24.6054) construction
  line L2022 (64.9111, 24.6054) -> (65.0755, 24.5828) construction
  line L2023 (65.0755, 24.5828) -> (65.24, 24.5593) construction
  line L2024 (65.24, 24.5593) -> (65.4046, 24.535) construction
  line L2025 (65.4046, 24.535) -> (65.5692, 24.5098) construction
  line L2026 (65.5692, 24.5098) -> (65.734, 24.4839) construction
  line L2027 (65.734, 24.4839) -> (65.8987, 24.4571) construction
  line L2028 (65.8987, 24.4571) -> (66.0636, 24.4294) construction
  line L2029 (66.0636, 24.4294) -> (66.2285, 24.401) construction
  line L2030 (66.2285, 24.401) -> (66.3935, 24.3718) construction
  line L2031 (66.3935, 24.3718) -> (66.5585, 24.3417) construction
  line L2032 (66.5585, 24.3417) -> (66.7236, 24.3108) construction
  line L2033 (66.7236, 24.3108) -> (66.8887, 24.2792) construction
  line L2034 (66.8887, 24.2792) -> (67.0208, 24.2532) construction
  line L2035 (67.0208, 24.2532) -> (67.1199, 24.2334) construction
  line L2036 (67.1199, 24.2334) -> (67.186, 24.22) construction
  line L2037 (67.186, 24.22) -> (67.2191, 24.2132) construction
  line L2038 (13.3622, -59.5542) -> (13.369, -59.5843) construction
  line L2039 (13.369, -59.5843) -> (13.3833, -59.6444) construction
  line L2040 (13.3833, -59.6444) -> (13.4071, -59.7338) construction
  line L2041 (13.4071, -59.7338) -> (13.4435, -59.8517) construction
  line L2042 (13.4435, -59.8517) -> (13.4951, -59.9973) construction
  line L2043 (13.4951, -59.9973) -> (13.5511, -60.1416) construction
  line L2044 (13.5511, -60.1416) -> (13.6099, -60.2852) construction
  line L2045 (13.6099, -60.2852) -> (13.6701, -60.4283) construction
  line L2046 (13.6701, -60.4283) -> (13.7313, -60.5711) construction
  line L2047 (13.7313, -60.5711) -> (13.7935, -60.7136) construction
  line L2048 (13.7935, -60.7136) -> (13.8571, -60.8557) construction
  line L2049 (13.8571, -60.8557) -> (13.9226, -60.9971) construction
  line L2050 (13.9226, -60.9971) -> (13.9902, -61.1379) construction
  line L2051 (13.9902, -61.1379) -> (14.06, -61.2779) construction
  line L2052 (14.06, -61.2779) -> (14.1316, -61.4173) construction
  line L2053 (14.1316, -61.4173) -> (14.205, -61.5561) construction
  line L2054 (14.205, -61.5561) -> (14.2797, -61.6944) construction
  line L2055 (14.2797, -61.6944) -> (14.3557, -61.8322) construction
  line L2056 (14.3557, -61.8322) -> (14.4327, -61.9697) construction
  line L2057 (14.4327, -61.9697) -> (14.5109, -62.1067) construction
  line L2058 (14.5109, -62.1067) -> (14.5904, -62.2432) construction
  line L2059 (14.5904, -62.2432) -> (14.6711, -62.3792) construction
  line L2060 (14.6711, -62.3792) -> (14.753, -62.5148) construction
  line L2061 (14.753, -62.5148) -> (14.8363, -62.6498) construction
  line L2062 (14.8363, -62.6498) -> (14.9208, -62.7843) construction
  line L2063 (14.9208, -62.7843) -> (15.0064, -62.9184) construction
  line L2064 (15.0064, -62.9184) -> (15.0932, -63.052) construction
  line L2065 (15.0932, -63.052) -> (15.181, -63.1852) construction
  line L2066 (15.181, -63.1852) -> (15.2698, -63.318) construction
  line L2067 (15.2698, -63.318) -> (15.3597, -63.4503) construction
  line L2068 (15.3597, -63.4503) -> (15.4506, -63.5821) construction
  line L2069 (15.4506, -63.5821) -> (15.5425, -63.7135) construction
  line L2070 (15.5425, -63.7135) -> (15.6354, -63.8445) construction
  line L2071 (15.6354, -63.8445) -> (15.7293, -63.975) construction
  line L2072 (15.7293, -63.975) -> (15.8242, -64.105) construction
  line L2073 (15.8242, -64.105) -> (15.92, -64.2346) construction
  line L2074 (15.92, -64.2346) -> (16.0168, -64.3638) construction
  line L2075 (16.0168, -64.3638) -> (16.1146, -64.4926) construction
  line L2076 (16.1146, -64.4926) -> (16.2132, -64.6209) construction
  line L2077 (16.2132, -64.6209) -> (16.3127, -64.7488) construction
  line L2078 (16.3127, -64.7488) -> (16.4131, -64.8762) construction
  line L2079 (16.4131, -64.8762) -> (16.5144, -65.0032) construction
  line L2080 (16.5144, -65.0032) -> (16.6166, -65.1298) construction
  line L2081 (16.6166, -65.1298) -> (16.7196, -65.256) construction
  line L2082 (16.7196, -65.256) -> (16.8235, -65.3817) construction
  line L2083 (16.8235, -65.3817) -> (16.9283, -65.507) construction
  line L2084 (16.9283, -65.507) -> (17.0338, -65.6318) construction
  line L2085 (17.0338, -65.6318) -> (17.1402, -65.7562) construction
  line L2086 (17.1402, -65.7562) -> (17.2474, -65.8802) construction
  line L2087 (17.2474, -65.8802) -> (17.3555, -66.0038) construction
  line L2088 (17.3555, -66.0038) -> (17.4643, -66.1269) construction
  line L2089 (17.4643, -66.1269) -> (17.5739, -66.2497) construction
  line L2090 (17.5739, -66.2497) -> (17.6842, -66.3719) construction
  line L2091 (17.6842, -66.3719) -> (17.7954, -66.4938) construction
  line L2092 (17.7954, -66.4938) -> (17.9073, -66.6152) construction
  line L2093 (17.9073, -66.6152) -> (18.02, -66.7362) construction
  line L2094 (18.02, -66.7362) -> (18.1335, -66.8568) construction
  line L2095 (18.1335, -66.8568) -> (18.2477, -66.9769) construction
  line L2096 (18.2477, -66.9769) -> (18.3626, -67.0966) construction
  line L2097 (18.3626, -67.0966) -> (18.4782, -67.2159) construction
  line L2098 (18.4782, -67.2159) -> (18.5946, -67.3347) construction
  line L2099 (18.5946, -67.3347) -> (18.7118, -67.4531) construction
  line L2100 (18.7118, -67.4531) -> (18.8296, -67.5711) construction
  line L2101 (18.8296, -67.5711) -> (18.9481, -67.6887) construction
  line L2102 (18.9481, -67.6887) -> (19.0674, -67.8058) construction
  line L2103 (19.0674, -67.8058) -> (19.1873, -67.9225) construction
  line L2104 (19.1873, -67.9225) -> (19.3079, -68.0388) construction
  line L2105 (19.3079, -68.0388) -> (19.4293, -68.1546) construction
  line L2106 (19.4293, -68.1546) -> (19.5512, -68.27) construction
  line L2107 (19.5512, -68.27) -> (19.6739, -68.385) construction
  line L2108 (19.6739, -68.385) -> (19.7726, -68.4767) construction
  line L2109 (19.7726, -68.4767) -> (19.8469, -68.5452) construction
  line L2110 (19.8469, -68.5452) -> (19.8966, -68.5908) construction
  line L2111 (19.8966, -68.5908) -> (19.9215, -68.6136) construction
  line L2112 (40.3263, -45.8153) -> (40.3467, -45.8385) construction
  line L2113 (40.3467, -45.8385) -> (40.3868, -45.8854) construction
  line L2114 (40.3868, -45.8854) -> (40.4451, -45.9573) construction
  line L2115 (40.4451, -45.9573) -> (40.5192, -46.056) construction
  line L2116 (40.5192, -46.056) -> (40.6066, -46.1833) construction
  line L2117 (40.6066, -46.1833) -> (40.6904, -46.3135) construction
  line L2118 (40.6904, -46.3135) -> (40.772, -46.4454) construction
  line L2119 (40.772, -46.4454) -> (40.8524, -46.5782) construction
  line L2120 (40.8524, -46.5782) -> (40.932, -46.7117) construction
  line L2121 (40.932, -46.7117) -> (41.0107, -46.8458) construction
  line L2122 (41.0107, -46.8458) -> (41.0883, -46.9807) construction
  line L2123 (41.0883, -46.9807) -> (41.1642, -47.1168) construction
  line L2124 (41.1642, -47.1168) -> (41.2383, -47.2543) construction
  line L2125 (41.2383, -47.2543) -> (41.3106, -47.393) construction
  line L2126 (41.3106, -47.393) -> (41.3813, -47.5329) construction
  line L2127 (41.3813, -47.5329) -> (41.4504, -47.6738) construction
  line L2128 (41.4504, -47.6738) -> (41.5184, -47.8156) construction
  line L2129 (41.5184, -47.8156) -> (41.5853, -47.9581) construction
  line L2130 (41.5853, -47.9581) -> (41.6512, -48.1012) construction
  line L2131 (41.6512, -48.1012) -> (41.716, -48.245) construction
  line L2132 (41.716, -48.245) -> (41.7798, -48.3895) construction
  line L2133 (41.7798, -48.3895) -> (41.8424, -48.5347) construction
  line L2134 (41.8424, -48.5347) -> (41.9039, -48.6807) construction
  line L2135 (41.9039, -48.6807) -> (41.9642, -48.8274) construction
  line L2136 (41.9642, -48.8274) -> (42.0234, -48.9749) construction
  line L2137 (42.0234, -48.9749) -> (42.0815, -49.123) construction
  line L2138 (42.0815, -49.123) -> (42.1386, -49.2717) construction
  line L2139 (42.1386, -49.2717) -> (42.1947, -49.421) construction
  line L2140 (42.1947, -49.421) -> (42.2499, -49.5709) construction
  line L2141 (42.2499, -49.5709) -> (42.3041, -49.7214) construction
  line L2142 (42.3041, -49.7214) -> (42.3574, -49.8724) construction
  line L2143 (42.3574, -49.8724) -> (42.4097, -50.024) construction
  line L2144 (42.4097, -50.024) -> (42.461, -50.1761) construction
  line L2145 (42.461, -50.1761) -> (42.5114, -50.3288) construction
  line L2146 (42.5114, -50.3288) -> (42.5608, -50.482) construction
  line L2147 (42.5608, -50.482) -> (42.6094, -50.6358) construction
  line L2148 (42.6094, -50.6358) -> (42.657, -50.79) construction
  line L2149 (42.657, -50.79) -> (42.7037, -50.9447) construction
  line L2150 (42.7037, -50.9447) -> (42.7495, -51.0999) construction
  line L2151 (42.7495, -51.0999) -> (42.7945, -51.2556) construction
  line L2152 (42.7945, -51.2556) -> (42.8386, -51.4118) construction
  line L2153 (42.8386, -51.4118) -> (42.8818, -51.5684) construction
  line L2154 (42.8818, -51.5684) -> (42.9241, -51.7255) construction
  line L2155 (42.9241, -51.7255) -> (42.9656, -51.883) construction
  line L2156 (42.9656, -51.883) -> (43.0063, -52.0409) construction
  line L2157 (43.0063, -52.0409) -> (43.0461, -52.1993) construction
  line L2158 (43.0461, -52.1993) -> (43.085, -52.3581) construction
  line L2159 (43.085, -52.3581) -> (43.1231, -52.5173) construction
  line L2160 (43.1231, -52.5173) -> (43.1604, -52.6769) construction
  line L2161 (43.1604, -52.6769) -> (43.1969, -52.8369) construction
  line L2162 (43.1969, -52.8369) -> (43.2326, -52.9973) construction
  line L2163 (43.2326, -52.9973) -> (43.2674, -53.1581) construction
  line L2164 (43.2674, -53.1581) -> (43.3015, -53.3193) construction
  line L2165 (43.3015, -53.3193) -> (43.3347, -53.4809) construction
  line L2166 (43.3347, -53.4809) -> (43.3672, -53.6428) construction
  line L2167 (43.3672, -53.6428) -> (43.3988, -53.8051) construction
  line L2168 (43.3988, -53.8051) -> (43.4297, -53.9677) construction
  line L2169 (43.4297, -53.9677) -> (43.4597, -54.1307) construction
  line L2170 (43.4597, -54.1307) -> (43.489, -54.294) construction
  line L2171 (43.489, -54.294) -> (43.5175, -54.4577) construction
  line L2172 (43.5175, -54.4577) -> (43.5453, -54.6217) construction
  line L2173 (43.5453, -54.6217) -> (43.5723, -54.7861) construction
  line L2174 (43.5723, -54.7861) -> (43.5984, -54.9508) construction
  line L2175 (43.5984, -54.9508) -> (43.6239, -55.1158) construction
  line L2176 (43.6239, -55.1158) -> (43.6486, -55.2811) construction
  line L2177 (43.6486, -55.2811) -> (43.6725, -55.4467) construction
  line L2178 (43.6725, -55.4467) -> (43.6956, -55.6126) construction
  line L2179 (43.6956, -55.6126) -> (43.718, -55.7789) construction
  line L2180 (43.718, -55.7789) -> (43.7397, -55.9454) construction
  line L2181 (43.7397, -55.9454) -> (43.7606, -56.1122) construction
  line L2182 (43.7606, -56.1122) -> (43.7767, -56.2459) construction
  line L2183 (43.7767, -56.2459) -> (43.7885, -56.3463) construction
  line L2184 (43.7885, -56.3463) -> (43.7962, -56.4133) construction
  line L2185 (43.7962, -56.4133) -> (43.8, -56.4469) construction
  line L2186 (13.3622, 59.5542) -> (13.369, 59.5843) construction
  line L2187 (13.369, 59.5843) -> (13.3833, 59.6444) construction
  line L2188 (13.3833, 59.6444) -> (13.4071, 59.7338) construction
  line L2189 (13.4071, 59.7338) -> (13.4435, 59.8517) construction
  line L2190 (13.4435, 59.8517) -> (13.4951, 59.9973) construction
  line L2191 (13.4951, 59.9973) -> (13.5511, 60.1416) construction
  line L2192 (13.5511, 60.1416) -> (13.6099, 60.2852) construction
  line L2193 (13.6099, 60.2852) -> (13.6701, 60.4283) construction
  line L2194 (13.6701, 60.4283) -> (13.7313, 60.5711) construction
  line L2195 (13.7313, 60.5711) -> (13.7935, 60.7136) construction
  line L2196 (13.7935, 60.7136) -> (13.8571, 60.8557) construction
  line L2197 (13.8571, 60.8557) -> (13.9226, 60.9971) construction
  line L2198 (13.9226, 60.9971) -> (13.9902, 61.1379) construction
  line L2199 (13.9902, 61.1379) -> (14.06, 61.2779) construction
  line L2200 (14.06, 61.2779) -> (14.1316, 61.4173) construction
  line L2201 (14.1316, 61.4173) -> (14.205, 61.5561) construction
  line L2202 (14.205, 61.5561) -> (14.2797, 61.6944) construction
  line L2203 (14.2797, 61.6944) -> (14.3557, 61.8322) construction
  line L2204 (14.3557, 61.8322) -> (14.4327, 61.9697) construction
  line L2205 (14.4327, 61.9697) -> (14.5109, 62.1067) construction
  line L2206 (14.5109, 62.1067) -> (14.5904, 62.2432) construction
  line L2207 (14.5904, 62.2432) -> (14.6711, 62.3792) construction
  line L2208 (14.6711, 62.3792) -> (14.753, 62.5148) construction
  line L2209 (14.753, 62.5148) -> (14.8363, 62.6498) construction
  line L2210 (14.8363, 62.6498) -> (14.9208, 62.7843) construction
  line L2211 (14.9208, 62.7843) -> (15.0064, 62.9184) construction
  line L2212 (15.0064, 62.9184) -> (15.0932, 63.052) construction
  line L2213 (15.0932, 63.052) -> (15.181, 63.1852) construction
  line L2214 (15.181, 63.1852) -> (15.2698, 63.318) construction
  line L2215 (15.2698, 63.318) -> (15.3597, 63.4503) construction
  line L2216 (15.3597, 63.4503) -> (15.4506, 63.5821) construction
  line L2217 (15.4506, 63.5821) -> (15.5425, 63.7135) construction
  line L2218 (15.5425, 63.7135) -> (15.6354, 63.8445) construction
  line L2219 (15.6354, 63.8445) -> (15.7293, 63.975) construction